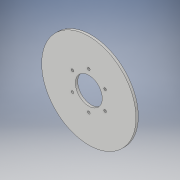
# Autodesk Inventor part: AZUSAsprocketbig
Saved by Autodesk Inventor 2019 (Build 230136000, 136)
## iProperties
Created: 2020-02-11
Part Number: AZUSAsprocketbig
Material: Generic
Document SubType Name: Modeling
Designer: rittmasm
Density: 1 g/cm^3
Appearance: Default
material_size: provided sprocket
Quantity: 1
Author: rittmasm
Autodesk Inventor part; units mm, degrees
ref_plane "YZ Plane" through (0, 0, 0) normal (1, 0, 0) x (0, 1, 0)
ref_plane "XZ Plane" through (0, 0, 0) normal (0, 1, 0) x (-1, 0, 0)
ref_plane "XY Plane" through (0, 0, 0) normal (0, 0, 1) x (1, 0, 0)
sketch "Sketch1" plane through (0, 0, 0) normal (0, 0, 1) x (1, 0, 0)
  circle A0 centre (0, 0) radius 36.195
  circle A1 centre (0, 0) radius 127
  dimension "d0" = 72.39
  dimension "d1" = 254
  constraints: 2 centre point, 2 coincident
  measures "d0" diameter of A0
  measures "d1" diameter of A1
extrude "Extrusion1" add sketch "Sketch1" along normal blind 6.35
sketch "Sketch3" plane through (0, 0, 6.35) normal (0, 0, 1) x (1, 0, 0)
  circle A0 centre (0, 0) radius 50.8
  circle A1 centre (0, 50.8) radius 3.3782
  circle A2 centre (-43.9941, 25.4) radius 3.3782
  circle A3 centre (-43.9941, -25.4) radius 3.3782
  circle A4 centre (0, -50.8) radius 3.3782
  circle A5 centre (43.9941, -25.4) radius 3.3782
  circle A6 centre (43.9941, 25.4) radius 3.3782
  dimension "d13" = 101.6
  dimension "d14" = 6.7564
  dimension "d17" = 360
  constraints: 6 centre point, 1 coincident, 1 vertical alignment, 15 other
  measures "d14" diameter of A1
extrude "Extrusion3" cut sketch "Sketch3" against normal blind 6.35 contours A6 A0 | A0 A6 | A5 A0 | A0 A5 | A1 A0 | A0 A1 | A4 A0 | A0 A4 | A2 A0 | A0 A2 | A3 A0 | A0 A3
body "Solid1"
